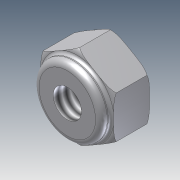
# Autodesk Inventor part: HW-00071
Saved by Autodesk Inventor 2012 (Build 160160000, 160)
## iProperties
Created: 2008-05-01
Part Number: HW-00071
Document SubType Name: Modeling
Designer: dfoster
Density: 1 g/cm^3
Description: Nut, Lock 10-24
Mass: 0.637638 g
Surface Area: 5.6464 cm^2
Volume: 0.637638 cm^3
Material: Default
Title: Nut, Lock 10-24
Author: dfoster
Autodesk Inventor part; units mm, degrees
ref_plane "YZ Plane" through (0, 0, 0) normal (1, 0, 0) x (0, 1, 0)
ref_plane "XZ Plane" through (0, 0, 0) normal (0, 1, 0) x (-1, 0, 0)
sketch "Sketch1" plane through (0, 0, 0) normal (0, 0, 1) x (1, 0, 0)
  line L0 (-12.7, 7.2007) -> (-17.4625, 9.9504)
  line L1 (-17.4625, 9.9504) -> (-17.4625, 15.4496)
  line L2 (-17.4625, 15.4496) -> (-12.7, 18.1993)
  line L3 (-12.7, 18.1993) -> (-7.9375, 15.4496)
  line L4 (-7.9375, 15.4496) -> (-7.9375, 9.9504)
  line L5 (-7.9375, 9.9504) -> (-12.7, 7.2007)
  point P0 (-12.7, 12.7)
  dimension "d0" = 9.525
  constraints: 12 end point, 13 other
  measures "d0" distance between parallel lines of L5 L2
extrude "Extrusion1" add sketch "Sketch1" along normal blind 4.6831
ref_plane "Work Plane1" through (-12.7, 18.1993, 4.6831) normal (-1, 0, 0) x (0, 0, -1)
sketch "Sketch3" plane through (-12.7, 18.1993, 4.6831) normal (-1, 0, 0) x (0, 0, -1)
  line L0 (0, 10.9985) -> (4.6831, 10.9985) projected
  line L1 (4.6831, 10.9985) -> (4.6831, 0) projected
  line L2 (4.6831, 0) -> (0, 0) projected
  line L3 (0, 0) -> (0, 10.9985) projected
  line L4 (0, 10.2365) -> (0, 5.4993)
  line L5 (0, 5.4993) -> (4.6831, 5.4993)
  line L6 (4.6831, 5.4993) -> (4.6831, 10.2365)
  arc A0 (4.6831, 10.2365) -> (4.3391, 10.9985) centre (3.6671, 10.2365) ccw
  arc A1 (0.344, 10.9985) -> (0, 10.2365) centre (1.016, 10.2365) ccw
  line L7 (0.344, 10.9985) -> (4.3391, 10.9985)
  line L8 (4.6831, 10.9985) -> (4.6831, 8.2489) projected
  line L9 (0, 10.9985) -> (0, 8.2489) projected
  line L10 (0, 8.2489) -> (0, 2.7496) projected
  dimension "d4" = 1.016
  dimension "d5" = 0.762
  dimension "d6" = 0.762
  constraints: 8 end point, 4 point on circle, 3 collinear, 2 centre point, 2 horizontal, 2 tangent, 1 equal radius, 1 midpoint, 1 perpendicular, 1 point on line, 1 vertical
  measures "d4" radius of A1
  measures "d5" distance from line of A1.centre L7
  measures "d6" distance from line of L7 A0.centre
revolve "Revolution1" cut sketch "Sketch3" angle 360 about axis through (-12.7, 12.7, 4.6831) along (0, 0, -1) keep common part contours L0 A0 L1 L5 L3 A1
sketch "Sketch4" plane through (0, 0, 4.6831) normal (0, 0, 1) x (1, 0, 0)
  circle A0 centre (-12.7, 12.7) radius 4.7373 projected
  circle A1 centre (-12.7, 12.7) radius 4.445
  point P0 (-16.3838, 16.989)
  point P1 (-18.2562, 13.7458)
  dimension "d8" = 8.89
  constraints: 1 centre point, 2 other
  measures "d8" diameter of A1
extrude "Extrusion2" add sketch "Sketch4" along normal blind 1.27 contours A1
fillet "Fillet1" radius 0.762 1 edges at (-17.145, 12.7, 5.9531)
fillet "Fillet2" radius 0.381 1 edges at (-17.145, 12.7, 4.6831)
hole "Hole1" at (-12.7, 12.7, 5.9531) direction (0, 0, -1) diameter 3.683 end through all thread size "10-24 UNC" class "2B" standard "ANSI Unified Screw Threads"
body "Solid1"
